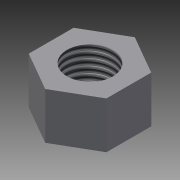
# Autodesk Inventor part: EEThreadedRodNut
Saved by Autodesk Inventor 2015 (Build 190159000, 159)
## iProperties
Created: 2017-01-14
Part Number: EEThreadedRodNut
Material: Generic
Document SubType Name: Modeling
Designer: 1esh9
Density: 1 g/cm^3
Appearance: Default
Author: 1esh9
Autodesk Inventor part; units mm, degrees
ref_plane "YZ Plane" through (0, 0, 0) normal (1, 0, 0) x (0, 1, 0)
ref_plane "XZ Plane" through (0, 0, 0) normal (0, 1, 0) x (-1, 0, 0)
ref_plane "XY Plane" through (0, 0, 0) normal (0, 0, 1) x (1, 0, 0)
sketch "Sketch1" plane through (0, 0, 0) normal (0, 0, 1) x (1, 0, 0)
  circle A0 centre (0, 0) radius 4.435
  line L0 (0, 8.6603) -> (7.5, 4.3301)
  line L1 (7.5, 4.3301) -> (7.5, -4.3301)
  line L2 (7.5, -4.3301) -> (0, -8.6603)
  line L3 (0, -8.6603) -> (-7.5, -4.3301)
  line L4 (-7.5, -4.3301) -> (-7.5, 4.3301)
  line L5 (-7.5, 4.3301) -> (0, 8.6603)
  dimension "d0" = 8.87
  dimension "d3" = 15
  constraints: 12 end point, 2 coincident, 1 centre point, 13 other
  measures "d0" diameter of A0
  measures "d3" distance between parallel lines of L4 L1
extrude "Extrusion1" add sketch "Sketch1" along normal blind 9
thread "Thread1" size "M9x1.25" class "6H" standard "ANSI Metric M Profile" full length
body "Solid1"
